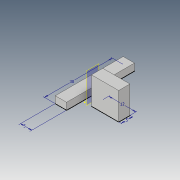
# Autodesk Inventor part: Incastri 1
Saved by Autodesk Inventor 2019 (Build 230136000, 136)
## iProperties
Created: 2019-06-02
Part Number: Incastri 1
Material: Generic
Document SubType Name: Modeling
Designer: giacomo
Density: 1 g/cm^3
Appearance: Default
Author: giacomo
Autodesk Inventor part; units mm, degrees
ref_plane "YZ Plane" through (0, 0, 0) normal (1, 0, 0) x (0, 1, 0)
ref_plane "XZ Plane" through (0, 0, 0) normal (0, 1, 0) x (-1, 0, 0)
ref_plane "XY Plane" through (0, 0, 0) normal (0, 0, 1) x (1, 0, 0)
sketch "Sketch1" plane through (0, 0, 0) normal (0, 1, 0) x (-1, 0, 0)
  line L0 (6, 7) -> (1, 7)
  line L1 (1, 7) -> (1, -23)
  line L2 (1, -23) -> (6, -23)
  line L3 (6, -23) -> (6, 7)
  line L4 (-3, 0) -> (-15, 0)
  line L5 (-15, 0) -> (-15, -5)
  line L6 (-15, -5) -> (-3, -5)
  line L7 (-3, -5) -> (-3, 0)
  point P0 (0, 0)
  dimension "d0" = 12
  dimension "d1" = 5
  dimension "d2" = 5
  dimension "d3" = 30
  constraints: 16 end point, 4 parallel, 2 horizontal, 2 perpendicular
  measures "d0" distance of L6.end L5.end
  measures "d1" distance of L5.end L4.end
  measures "d2" distance of L0.start L0.end
  measures "d3" distance of L2.end L0.start
extrude "Extrusion1" add sketch "Sketch1" along normal blind 3 contours L3 L2 L1 L0
extrude "Extrusion2" add sketch "Sketch1" along normal blind 12 contours L7 L6 L5 L4
ref_plane "Work Plane1" through (1, 0, -5) normal (-1, 0, 0) x (0, 0, 1)
split body "Split1" result two bodies by plane through (1, 0, -5) normal (-1, 0, 0) first body at (-4.3333, 0.5, -13)
body "Solid2"
body "Solid3"
